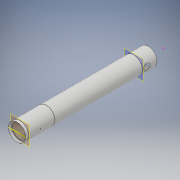
# Autodesk Inventor part: 塔体
Saved by Autodesk Inventor 2018.2 (Build 222227000, 227)
## iProperties
Created: 2018-07-04
Part Number: 塔体
Material: 常规
Document SubType Name: Modeling
Designer: Administrator
Density: 1 g/cm^3
Appearance: 默认
Author: Administrator
Autodesk Inventor part; units mm, degrees
ref_plane "YZ Plane" through (0, 0, 0) normal (1, 0, 0) x (0, 1, 0)
ref_plane "XZ Plane" through (0, 0, 0) normal (0, 1, 0) x (-1, 0, 0)
ref_plane "XY Plane" through (0, 0, 0) normal (0, 0, 1) x (1, 0, 0)
sketch "草图1" plane through (0, 0, 0) normal (0, 1, 0) x (-1, 0, 0)
  circle A0 centre (0, 0) radius 600
  line L0 (0, 600) -> (0, 520)
  circle A1 centre (0, 0) radius 520
  dimension "d0" = 1200
  dimension "d9" = 80
  constraints: 2 coincident, 2 end point, 2 vertical alignment, 1 vertical, 4 other
  measures "d9" distance of L0.start L0.end
surface extrude "拉伸曲面1" sketch "草图1" along normal blind 8000 shown no curves A0
thicken "加厚1" operation new thickness 3.7 both sides no extend neighbours no toward (0.9998154, 0, 0.0192135) faces at (-599.8892, 5333.3333, -11.5281)
ref_plane "工作平面5" through (0, 2000, 0) normal (0, 1, 0) x (-1, 0, 0)
sketch "草图3" plane through (0, 2000, 0) normal (0, 1, 0) x (-1, 0, 0)
  circle A0 centre (0, 0) radius 520 projected
  circle A1 centre (0, 0) radius 600 projected
extrude "拉伸1" add sketch "草图3" along normal blind 10
ref_plane "工作平面3" through (0, 200, 0) normal (0, -1, 0) x (1, 0, 0)
sketch "草图5" plane through (0, 200, 0) normal (0, -1, 0) x (1, 0, 0)
  circle A0 centre (0, 0) radius 520 projected
  circle A1 centre (0, 0) radius 596.3 projected
extrude "拉伸3" add sketch "草图5" along normal blind 10
sketch "草图6" plane through (0, 0, 0) normal (1, 0, 0) x (0, 1, 0)
  line L0 (0, 0) -> (1000, 0)
  circle A0 centre (1000, 0) radius 23.5
  dimension "d19" = 1000
  dimension "d20" = 47
  constraints: 2 end point, 1 centre point, 1 coincident, 1 horizontal
  measures "d19" distance of L0.start L0.end
  measures "d20" diameter of A0
extrude "拉伸4" cut sketch "草图6" along normal blind 1000
ref_plane "工作平面13" through (0, 10000, 0) normal (0, 1, 0) x (-1, 0, 0)
sketch "草图7" plane through (0, 10000, 0) normal (0, 1, 0) x (-1, 0, 0)
  point P0 (0, 0)
ref_plane "工作平面8" through (0, 8000, 0) normal (0, 1, 0) x (1, 0, 0)
sketch "草图10" plane through (0, 8000, 0) normal (0, 1, 0) x (1, 0, 0)
  circle A0 centre (0, 0) radius 520 projected
  circle A1 centre (0, 0) radius 596.3 projected
extrude "拉伸7" add sketch "草图10" against normal blind 10
sketch "草图11" plane through (0, 0, 0) normal (0, 0, 1) x (1, 0, 0)
  line L0 (-596.3, 2010) -> (596.3, 2010) projected
  line L1 (596.3, 0) -> (-596.3, 0) projected
  point P0 (0, 0)
sketch "草图12" plane through (0, 8000, 0) normal (0, 1, 0) x (1, 0, 0)
  circle A0 centre (0, 0) radius 600 projected
surface extrude "拉伸曲面2" sketch "草图12" along normal blind 1000 shown no curves A0
thicken "加厚2" operation add thickness 3.7 both sides no extend neighbours no toward (-0.9998154, 0, -0.0192135) faces at (599.8892, 8666.6667, 11.5281)
sketch "草图13" plane through (0, 0, 0) normal (1, 0, 0) x (0, 1, 0)
  line L0 (9000, -596.3) -> (9000, 596.3) projected
  line L1 (9000, 0) -> (8600, 0)
  line L2 (8600, 0) -> (8300, 0)
  circle A0 centre (8600, 0) radius 225
  circle A1 centre (8300, 0) radius 225
  point P0 (0, 0)
  dimension "d38" = 400
  dimension "d39" = 300
  dimension "d40" = 450
  dimension "d41" = 450
  constraints: 4 end point, 2 centre point, 2 coincident, 1 horizontal, 1 midpoint, 1 point on line
  measures "d38" distance of L1.start L1.end
  measures "d39" distance of L1.end L2.end
  measures "d40" diameter of A0
  measures "d41" diameter of A1
extrude "拉伸8" cut sketch "草图13" along normal blind 1000 contours A1 L2 A0 | A0 A1 | A0 L2 A1
extrude "拉伸9" cut sketch "草图13" against normal blind 1000 contours A0 A1 L2 L1 | L1 L2 A1 A0 | A1 L2 A0 | A0 L2 A1
sketch "草图14" plane through (0, 0, 0) normal (1, 0, 0) x (0, 1, 0)
  line L0 (8000, 520) -> (8000, -520) projected
  line L1 (8000, 0) -> (7400, 0)
  circle A0 centre (7400, 0) radius 225
  point P0 (0, 0)
  dimension "d46" = 600
  dimension "d47" = 450
  constraints: 2 end point, 1 centre point, 1 coincident, 1 horizontal, 1 midpoint
  measures "d46" distance of L1.start L1.end
  measures "d47" diameter of A0
extrude "拉伸10" cut sketch "草图14" against normal blind 1000
sketch "草图15" plane through (0, 0, 0) normal (1, 0, 0) x (0, 1, 0)
  line L0 (2010, 596.3) -> (2010, -596.3) projected
  line L1 (2010, 0) -> (1610, 0)
  circle A0 centre (1610, 0) radius 225
  point P0 (0, 0)
  dimension "d50" = 400
  dimension "d51" = 450
  constraints: 2 end point, 1 centre point, 1 coincident, 1 horizontal, 1 midpoint
  measures "d50" distance of L1.start L1.end
  measures "d51" diameter of A0
extrude "拉伸11" cut sketch "草图15" against normal blind 1000
sketch "草图16" plane through (0, 0, 0) normal (0, 0, 1) x (1, 0, 0)
  line L0 (596.3, 9000) -> (-596.3, 9000) projected
  line L1 (0, 9000) -> (0, 8700)
  line L2 (0, 8700) -> (0, 8500)
  line L3 (0, 8500) -> (0, 8300)
  circle A0 centre (0, 8700) radius 15
  circle A1 centre (0, 8500) radius 15
  circle A2 centre (0, 8300) radius 15
  point P0 (0, 0)
  dimension "d54" = 300
  dimension "d55" = 200
  dimension "d56" = 200
  dimension "d57" = 30
  dimension "d58" = 30
  dimension "d59" = 30
  constraints: 6 end point, 3 centre point, 3 coincident, 2 point on line, 1 midpoint, 1 vertical
  measures "d54" distance of L1.start L1.end
  measures "d55" distance of L1.end L2.end
  measures "d56" distance of L2.end L3.end
  measures "d57" diameter of A0
  measures "d58" diameter of A1
  measures "d59" diameter of A2
extrude "拉伸12" cut sketch "草图16" against normal blind 1000
body "Srf1"
body "Srf2"
